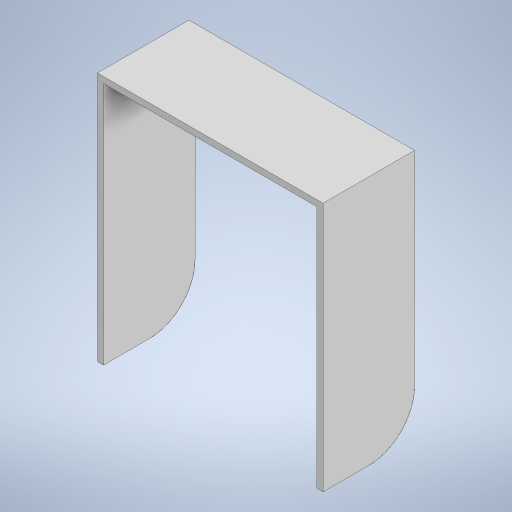
# Autodesk Inventor part: выступ АКБ
Saved by Autodesk Inventor 2023.1 (Build 271208000, 208)
## iProperties
Created: 2023-04-15
Part Number: выступ АКБ
Material: Типовые
Document SubType Name: Modeling
Designer: User
Density: 1 g/cm^3
Appearance: По умолчанию
Author: User
Autodesk Inventor part; units mm, degrees
ref_plane "YZ Plane" through (0, 0, 0) normal (1, 0, 0) x (0, 1, 0)
ref_plane "XZ Plane" through (0, 0, 0) normal (0, 1, 0) x (-1, 0, 0)
ref_plane "XY Plane" through (0, 0, 0) normal (0, 0, 1) x (1, 0, 0)
sketch "Эскиз1" plane through (0, 0, 0) normal (0, 0, 1) x (1, 0, 0)
  line L0 (-37, 0) -> (37, 0)
  line L1 (37, 0) -> (37, 82)
  line L2 (37, 82) -> (-37, 82)
  line L3 (-37, 82) -> (-37, 0)
  line L4 (-35, 0) -> (35, 0)
  line L5 (35, 0) -> (35, 80)
  line L6 (35, 80) -> (-35, 80)
  line L7 (-35, 80) -> (-35, 0)
  line L8 (0, -16.4) -> (0, 98.4) projected
  point P0 (0, 0)
  dimension "d0" = 70
  dimension "d1" = 80
  dimension "d2" = 2
  dimension "d3" = 2
  dimension "d4" = 2
  constraints: 16 end point, 4 parallel, 2 horizontal, 2 perpendicular, 1 point on line, 2 other
  measures "d0" distance between parallel lines of L5 L7
  measures "d1" distance between parallel lines of L0 L6
  measures "d2" distance between parallel lines of L7 L3
  measures "d3" distance between parallel lines of L6 L2
  measures "d4" distance between parallel lines of L1 L5
extrude "Выдавливание1" add sketch "Эскиз1" along normal blind 30 contours L3 L2 L8 L6 L7 L0 | L2 L1 L0 L5 L6 L8
fillet "Сопряжение1" radius 15 2 edges at (36, 0, 0) (-36, 0, 0)
